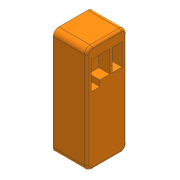
# Autodesk Inventor part: U2D2
Saved by Autodesk Inventor 2019.4 (Build 234330000, 330)
## iProperties
Created: 2018-05-25
Part Number: U2D2
Material: ABS プラスチック
Document SubType Name: Modeling
Designer: student
Density: 1.06 g/cm^3
Appearance: 滑らか - 黄
Mass: 12.7514 g
Surface Area: 40.9392 cm^2
Volume: 12.0296 cm^3
Sending System: SolidWorks 2017
Last Author: y6tada
Last Saved: 2018-06-10
Author: student
Autodesk Inventor part; units mm, degrees
ref_plane "YZ Plane" through (0, 0, 0) normal (1, 0, 0) x (0, 1, 0)
ref_plane "XZ Plane" through (0, 0, 0) normal (0, 1, 0) x (-1, 0, 0)
ref_plane "XY Plane" through (0, 0, 0) normal (0, 0, 1) x (1, 0, 0)
sketch "スケッチ2" plane through (0, -6.5, -24) normal (-1, 0, 0) x (0, 0, 1)
  arc A0 (2.5, 15.5) -> (0, 13) centre (2.5, 13) ccw projected
  line L0 (0, 0) -> (0, 13) projected
  arc A1 (0, 0) -> (2.5, -2.5) centre (2.5, 0) ccw projected
  line L1 (45.5, -2.5) -> (2.5, -2.5) projected
  arc A2 (45.5, -2.5) -> (48, 0) centre (45.5, 0) ccw projected
  line L2 (48, 13) -> (48, 0) projected
  arc A3 (48, 13) -> (45.5, 15.5) centre (45.5, 13) ccw projected
  line L3 (2.5, 15.5) -> (45.5, 15.5) projected
  point P0 (24, 6.5)
extrude "押し出し2" add sketch "スケッチ2" along normal blind 15
sketch "スケッチ1" plane through (-15, -6.5, -24) normal (-1, 0, 0) x (0, 0, 1)
  line L0 (24, 6.5) -> (24, -15.1868) construction
  circle A0 centre (45, 6.5) radius 0.8
  circle A1 centre (3, 6.5) radius 0.8
  line L1 (45, 6.5) -> (24, 6.5) construction
  dimension "d0" = 1.6
  dimension "d1" = 42
  constraints: 4 end point, 2 centre point, 1 equal radius, 1 horizontal, 1 symmetric about line, 1 vertical, 1 other
  measures "d0" diameter of A0
  measures "d1" diameter of L1.start L0
extrude "押し出し1" cut sketch "スケッチ1" against normal blind 5.5
sketch "スケッチ3" plane through (0, -6.5, -24) normal (-1, 0, 0) x (0, 0, -1)
  line L0 (-33.2, -7.925) -> (-43, -7.925)
  line L1 (-43, -7.925) -> (-43, 0.425)
  line L2 (-43, 0.425) -> (-30.55, 0.425)
  line L3 (-30.55, 0.425) -> (-30.55, -3.425)
  line L4 (-30.55, -3.425) -> (-33.2, -3.425)
  line L5 (-33.2, -3.425) -> (-33.2, -7.925)
  line L6 (-43, -13.425) -> (-43, -8.925)
  line L7 (-43, -8.925) -> (-33.2, -8.925)
  line L8 (-33.2, -8.925) -> (-33.2, -13.425)
  line L9 (-33.2, -13.425) -> (-43, -13.425)
  point P0 (-24, -6.5)
  constraints: 20 end point
extrude "押し出し3" cut sketch "スケッチ3" along normal blind 5
fillet "フィレット1" radius 1 8 edges at (0, 8.2678, -23.2678) (0, 0, -24) (0, -8.2678, -23.2678) (0, -9, 0) (0, -8.2678, 23.2678) (0, 0, 24) (0, 8.2678, 23.2678) (0, 9, 0)
sketch "スケッチ4" plane through (-15, -6.5, -24) normal (0, 0, -1) x (-1, 0, 0)
  line L0 (-11.15, 2.5) -> (-8.15, 2.5)
  line L1 (-8.15, 2.5) -> (-8.15, 10.5)
  line L2 (-8.15, 10.5) -> (-11.15, 10.5)
  line L3 (-11.15, 10.5) -> (-11.15, 2.5)
  line L4 (-15, 6.5) -> (-11.15, 6.5) construction
  dimension "d9" = 8
  dimension "d10" = 3
  dimension "d11" = 3.85
  constraints: 10 end point, 2 horizontal, 2 parallel, 1 midpoint, 1 perpendicular
  measures "d9" distance of L0.end L1.end
  measures "d10" distance of L1.end L2.end
  measures "d11" distance of L4.start L4.end
extrude "押し出し4" cut sketch "スケッチ4" against normal blind 5
